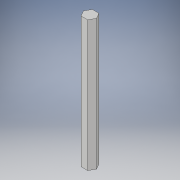
# Autodesk Inventor part: 6x10inAxleV1
Saved by Autodesk Inventor 2019 (Build 230136000, 136)
## iProperties
Created: 2021-09-16
Part Number: 6x10inAxleV1
Material: Generic
Document SubType Name: Modeling
Designer: timmy
Density: 1 g/cm^3
Appearance: Default
Author: timmy
Autodesk Inventor part; units mm, degrees
ref_plane "YZ Plane" through (0, 0, 0) normal (1, 0, 0) x (0, 1, 0)
ref_plane "XZ Plane" through (0, 0, 0) normal (0, 1, 0) x (-1, 0, 0)
ref_plane "XY Plane" through (0, 0, 0) normal (0, 0, 1) x (1, 0, 0)
sketch "Sketch1" plane through (0, 0, 0) normal (0, 1, 0) x (-1, 0, 0)
  line L0 (0, 0) -> (12.7, 0)
  line L1 (12.7, 0) -> (6.35, -10.9985)
  line L2 (6.35, -10.9985) -> (-6.35, -10.9985)
  line L3 (-6.35, -10.9985) -> (-12.7, 0)
  line L4 (-12.7, 0) -> (-6.35, 10.9985)
  line L5 (-6.35, 10.9985) -> (6.35, 10.9985)
  line L6 (6.35, 10.9985) -> (12.7, 0)
  dimension "d0" = 12.7
  constraints: 14 end point, 1 coincident, 1 horizontal, 13 other
  measures "d0" distance of L0.start L0.end
extrude "Extrusion1" add sketch "Sketch1" along normal blind 254
body "Solid1"
